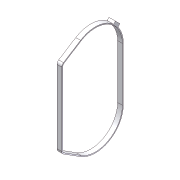
# Autodesk Inventor part: battery_cord_2x
Saved by Autodesk Inventor 2014 SP1 (Build 180222100, 222)
## iProperties
Created: 2012-08-10
Part Number: battery_cord_2x
Document SubType Name: Modeling
Designer: Robert Davis
Density: 0.1 g/cm^3
Material: Polyester Yarn
Mass: 0.00453414 g
Surface Area: 3.62733 cm^2
Volume: 0.0453414 cm^3
Appearance: Smooth - White
Author: Robert Davis
Autodesk Inventor part; units mm, degrees
ref_plane "YZ Plane" through (0, 0, 0) normal (1, 0, 0) x (0, 1, 0)
ref_plane "XZ Plane" through (0, 0, 0) normal (0, 1, 0) x (-1, 0, 0)
ref_plane "XY Plane" through (0, 0, 0) normal (0, 0, 1) x (1, 0, 0)
sketch "Sketch1" plane through (0, 0, 0) normal (0, 0, 1) x (1, 0, 0)
  line L0 (-0.75, 0.15) -> (0.75, 0.15)
  line L1 (0.75, 0.15) -> (0.75, -0.15)
  line L2 (0.75, -0.15) -> (-0.75, -0.15)
  line L3 (-0.75, -0.15) -> (-0.75, 0.15)
  line L4 (0, -0.2204) -> (0, 0)
  line L5 (0, 0) -> (0.3288, 0)
  dimension "d0" = 1.5
  dimension "d1" = 0.3
  constraints: 12 end point, 2 horizontal, 2 vertical, 1 coincident, 2 other
  measures "d0" distance of L0.start L0.end
  measures "d1" distance of L0.end L1.end
sketch3d "3D Sketch1"
  line L0 (0, 0, 0) -> (0, 0, 11.4491)
  arc A0 (0, 0, 11.4491) -> (0, 0.4657, 12.2944) centre (0, 1, 11.4491) ccw
  line L1 (0, 0.4657, 12.2944) -> (0, 5.8049, 15.6693)
  arc A1 (0, 5.8049, 15.6693) -> (0, 19, 8.4) centre (0, 10.4, 8.3999) ccw
  line L2 (0, 19, 8.4) -> (0, 19, -8.4)
  arc A2 (0, 19, -8.4) -> (0, 5.8048, -15.6694) centre (0, 10.4, -8.4) ccw
  line L3 (0, 5.8048, -15.6694) -> (0, 0.4657, -12.2944)
  arc A3 (0, 0.4657, -12.2944) -> (0, 0, -11.4491) centre (0, 1, -11.4491) ccw
  line L4 (0, 0, -11.4491) -> (0, 0, 0)
  dimension "d10" = 16.8
  dimension "d11" = 12
  dimension "d12" = 12
  dimension "d13" = 19
  dimension "d2" = 8.6
  dimension "d3" = 8.6
  dimension "d5" = 1
  dimension "d6" = 1
  constraints: 20 horizontal
sweep "Sweep1" add profiles "Sketch1" path "3D Sketch1"
sketch "Sketch2" plane through (0, 0, 0) normal (1, 0, 0) x (0, 1, 0)
  line L0 (17.8246, 14.4103) -> (17.1175, 13.7032)
  line L1 (17.1175, 13.7032) -> (15.7033, 15.1174)
  line L2 (15.7033, 15.1174) -> (16.4104, 15.8245)
  line L3 (16.4104, 15.8245) -> (17.8246, 14.4103)
  arc A0 (18.85, 8.4) -> (5.8851, 15.5425) centre (10.4, 8.3999) ccw projected
  line L4 (10.4, 8.3999) -> (24.1814, 22.1813) construction
  line L5 (-0.15, -11.4491) -> (-0.15, 11.4491) construction
  point P0 (0, 0)
  point P1 (16.4104, 14.4103)
  point P2 (16.4104, 14.4103)
  dimension "d15" = 2
  dimension "d16" = 1
  dimension "d17" = 45
  dimension "d18" = 8.5
  constraints: 10 end point, 2 coincident, 2 parallel, 2 perpendicular, 1 midpoint, 1 point on line
  measures "d15" distance of L2.end L0.start
  measures "d16" distance of L1.end L2.end
  measures "d17" angle of L5 L4
  measures "d18" distance of A0.centre point (16.41, 14.41)
extrude "Extrusion1" add sketch "Sketch2" along normal mid plane 2
equation "\"d6\" = d5"
body "Solid1"
